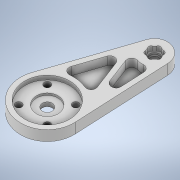
# Autodesk Inventor part: 足首_独立ピッチ_1_1
Saved by Autodesk Inventor 2020 (Build 240168000, 168)
## iProperties
Created: 2021-09-01
Part Number: 足首_独立ピッチ_1_1
Material: アルミニウム 2014-T4
Document SubType Name: Modeling
Designer: naoki
Density: 2.8 g/cm^3
Appearance: 滑らか - 淡い灰色
Author: naoki
Autodesk Inventor part; units mm, degrees
ref_plane "YZ Plane" through (0, 0, 0) normal (1, 0, 0) x (0, 1, 0)
ref_plane "XZ Plane" through (0, 0, 0) normal (0, 1, 0) x (-1, 0, 0)
ref_plane "XY Plane" through (0, 0, 0) normal (0, 0, 1) x (1, 0, 0)
derived "下半身全体像_1_1.ipt"
sketch "スケッチ1" plane through (0, 0, 0) normal (0, 0, 1) x (1, 0, 0)
  circle A0 centre (0, 0) radius 10.5 construction
  line L0 (0, 0) -> (-12, 0) construction
  arc A1 (0, 16) -> (-12, 10.583) centre (0, 0) ccw construction
  arc A2 (-12, -10.583) -> (0, -16) centre (0, 0) ccw construction
  line L1 (0, 16) -> (39.5, 16) construction
  line L2 (39.5, 16) -> (39.5, -16) construction
  line L3 (39.5, -16) -> (0, -16) construction
  circle A3 centre (1, 13.5) radius 1.35 projected
  circle A4 centre (1, -13.5) radius 1.35 projected
  circle A5 centre (28, 13.5) radius 1.35 projected
  circle A6 centre (28, -13.5) radius 1.35 projected
  line L4 (1, 13.5) -> (1, -13.5) construction
  line L5 (1, -13.5) -> (28, -13.5) construction
  line L6 (1, 13.5) -> (28, 13.5) construction
  line L7 (28, 13.5) -> (28, -13.5) construction
  line L8 (0, 0) -> (1, 0) construction
  line L9 (32, 120) -> (32, 20) construction
  line L10 (0, 0) -> (0, 0) construction
  circle A7 centre (32, 120) radius 4.05 projected
  line L11 (0, 140) -> (0, 40) construction
  circle A8 centre (0, 40) radius 4.05 projected
  line L12 (0, 0) -> (0, -100) construction
  line L13 (32, 20) -> (32, -80) construction
  line L14 (0, 0) -> (0, 40) construction
  circle A9 centre (32, 20) radius 6.5 construction
  line L15 (32, 23.5218) -> (35.05, 21.7609) construction
  line L16 (35.05, 21.7609) -> (35.05, 18.2391) construction
  line L17 (35.05, 18.2391) -> (32, 16.4782) construction
  line L18 (32, 16.4782) -> (28.95, 18.2391) construction
  line L19 (28.95, 18.2391) -> (28.95, 21.7609) construction
  line L20 (28.95, 21.7609) -> (32, 23.5218) construction
  line L21 (21.5, 152) -> (61, 152) construction
  line L22 (61, 152) -> (61, 100.5) construction
  line L23 (61, 100.5) -> (21.5, 100.5) construction
  line L24 (21.5, 100.5) -> (21.5, 152) construction
  line L25 (21.5, 140) -> (61, 140) construction
  line L26 (16, 150.5) -> (66.5, 150.5) construction
  line L27 (66.5, 150.5) -> (66.5, 129.5) construction
  line L28 (66.5, 129.5) -> (16, 129.5) construction
  line L29 (16, 129.5) -> (16, 150.5) construction
  circle A10 centre (0, 140) radius 10.5 construction
  line L30 (-13.5, 139) -> (13.5, 139) construction
  line L31 (13.5, 139) -> (13.5, 112) construction
  line L32 (13.5, 112) -> (-13.5, 112) construction
  line L33 (-13.5, 112) -> (-13.5, 139) construction
  circle A11 centre (-13.5, 139) radius 1.35 projected
  circle A12 centre (13.5, 139) radius 1.35 projected
  circle A13 centre (-13.5, 112) radius 1.35 projected
  circle A14 centre (13.5, 112) radius 1.35 projected
  line L34 (-12, 10.583) -> (-12, -10.583) construction
  circle A15 centre (0, -100) radius 4.05 construction
  circle A16 centre (32, -80) radius 4.05 construction
  circle A17 centre (0, -100) radius 10.5 construction
  line L35 (32, -80) -> (0, -100) construction
  line L36 (45, -60.5) -> (77.5, -60.5) construction
  line L37 (77.5, -60.5) -> (77.5, -112) construction
  line L38 (77.5, -112) -> (45, -112) construction
  line L39 (45, -112) -> (45, -60.5) construction
  line L40 (45, -100) -> (77.5, -100) construction
  line L41 (39.5, -89.5) -> (83, -89.5) construction
  line L42 (83, -89.5) -> (83, -110.5) construction
  line L43 (83, -110.5) -> (39.5, -110.5) construction
  line L44 (39.5, -110.5) -> (39.5, -89.5) construction
  line L45 (1, -86.5) -> (28, -86.5) construction
  line L46 (28, -86.5) -> (28, -113.5) construction
  line L47 (28, -113.5) -> (1, -113.5) construction
  line L48 (1, -113.5) -> (1, -86.5) construction
  circle A18 centre (1, -86.5) radius 1.35 construction
  circle A19 centre (1, -113.5) radius 1.35 construction
  circle A20 centre (28, -113.5) radius 1.35 construction
  circle A21 centre (28, -86.5) radius 1.35 construction
  circle A22 centre (32, 20) radius 4.05 projected
  circle A23 centre (32, 20) radius 4.05 projected
  line L49 (10.583, 152) -> (-10.583, 152) construction
  line L50 (16, 140) -> (16, 100.5) construction
  line L51 (16, 100.5) -> (-16, 100.5) construction
  line L52 (-16, 100.5) -> (-16, 140) construction
  arc A24 (16, 140) -> (10.583, 152) centre (0, 140) ccw construction
  arc A25 (-10.583, 152) -> (-16, 140) centre (0, 140) ccw construction
  line L53 (-12, -89.417) -> (-12, -110.583) construction
  line L54 (0, -84) -> (39.5, -84) construction
  line L55 (39.5, -84) -> (39.5, -116) construction
  line L56 (39.5, -116) -> (0, -116) construction
  arc A26 (0, -84) -> (-12, -89.417) centre (0, -100) ccw construction
  arc A27 (-12, -110.583) -> (0, -116) centre (0, -100) ccw construction
  circle A28 centre (-8.5, 0) radius 1.35 projected
  circle A29 centre (0, 0) radius 8.5 construction
  line L57 (35.05, 121.7609) -> (35.05, 118.2391) construction
  line L58 (35.05, 118.2391) -> (32, 116.4782) construction
  line L59 (32, 116.4782) -> (28.95, 118.2391) construction
  line L60 (28.95, 118.2391) -> (28.95, 121.7609) construction
  line L61 (28.95, 121.7609) -> (32, 123.5218) construction
  line L62 (32, 123.5218) -> (35.05, 121.7609) construction
  line L63 (0, 152) -> (0, 140) construction
  line L64 (0, 140) -> (0, 139) construction
  circle A30 centre (0, -100) radius 5.01
  circle A31 centre (0, -100) radius 12 construction
  circle A32 centre (-8.5, -100) radius 1.35
  line L65 (-24.9932, -100) -> (93.0564, -100) construction
  circle A33 centre (0, -100) radius 2.25
  circle A34 centre (0, -100) radius 12.5
  circle A35 centre (0, -100) radius 10.51
  circle A36 centre (0, -108.5) radius 1.35
  circle A37 centre (8.5, -100) radius 1.35
  circle A38 centre (0, -91.5) radius 1.35
  circle A39 centre (32, -80) radius 1.55
  circle A40 centre (32, -80) radius 2.25
  line L66 (-4.7001, -88.4173) -> (29.7439, -74.4403)
  line L67 (36.0089, -84.4642) -> (8.3518, -109.3004)
  circle A41 centre (32, -80) radius 6
  circle A42 centre (32, -80) radius 2.76 construction
  line L68 (33.5935, -82.76) -> (32.5435, -82.76)
  line L69 (30.4065, -82.76) -> (29.8815, -81.8507)
  line L70 (28.813, -80) -> (29.338, -79.0907)
  line L71 (30.4065, -77.24) -> (31.4565, -77.24)
  line L72 (33.5935, -77.24) -> (35.187, -80)
  line L73 (35.187, -80) -> (33.5935, -82.76)
  arc A43 (31.4565, -77.24) -> (29.8815, -78.1493) centre (30.9315, -78.1493) ccw
  line L74 (32, -80) -> (30.4065, -77.24) construction
  arc A44 (29.338, -79.0907) -> (29.338, -80.9093) centre (29.863, -80) ccw
  arc A45 (29.8815, -81.8507) -> (31.4565, -82.76) centre (30.9315, -81.8507) ccw
  arc A46 (32.5435, -82.76) -> (34.1185, -81.8507) centre (33.0685, -81.8507) ccw
  arc A47 (34.662, -80.9093) -> (34.662, -79.0907) centre (34.137, -80) ccw
  arc A48 (34.1185, -78.1493) -> (32.5435, -77.24) centre (33.0685, -78.1493) ccw
  line L75 (31.3452, -85.9642) -> (12.0618, -103.2808)
  line L76 (2.3365, -87.7203) -> (26.352, -77.9751)
  line L77 (26.734, -77.1244) -> (26.2459, -78.0181) construction
  line L78 (12.825, -102.5953) -> (10.9709, -105.9909) construction
  line L79 (26.2459, -78.0181) -> (12.825, -102.5953)
  line L80 (23.3185, -79.2061) -> (12.4661, -99.0797)
  line L81 (31.4565, -77.24) -> (32.5435, -77.24)
  line L82 (32.5435, -77.24) -> (33.5935, -77.24)
  line L83 (29.8815, -78.1493) -> (30.4065, -77.24)
  line L84 (29.338, -79.0907) -> (29.8815, -78.1493)
  line L85 (29.338, -80.9093) -> (28.813, -80)
  line L86 (29.8815, -81.8507) -> (29.338, -80.9093)
  line L87 (31.4565, -82.76) -> (30.4065, -82.76)
  line L88 (32.5435, -82.76) -> (31.4565, -82.76)
  point P0 (66.5, 140)
  point P1 (39.5, 0)
  point P2 (83, -100)
  point P3 (1, -100)
  point P4 (-12, -100)
  point P5 (39.5, -100)
  point P6 (83, -100)
  point P7 (34.3902, -81.38)
  point P8 (28.813, -80)
  point P9 (30.4065, -82.76)
  point P10 (33.5935, -82.76)
  point P11 (35.187, -80)
  point P12 (33.5935, -77.24)
  point P13 (34.662, -80.9093)
  point P14 (34.662, -79.0907)
  point P15 (34.1185, -78.1493)
  dimension "d5" = 17
  dimension "d60" = 5.52
  dimension "d2" = 10.02
  dimension "d15" = 8.5
  dimension "d48" = 4.5
  dimension "d49" = 25
  dimension "d50" = 21.02
  dimension "d51" = 2.7
  dimension "d54" = 360
  dimension "d56" = 3.1
  dimension "d58" = 4.5
  dimension "d59" = 6
  dimension "d61" = 2.1
  dimension "d64" = 360
  dimension "d68" = 2
  dimension "d69" = 2
  dimension "d71" = 2
  constraints: 48 end point, 29 point on circle, 18 centre point, 12 coincident, 11 tangent, 6 parallel, 6 point on line, 2 horizontal, 2 midpoint, 1 horizontal alignment, 1 perpendicular, 1 vertical, 60 other
  measures "d2" diameter of A30
  measures "d15" distance of A32.centre A15.centre
  measures "d48" diameter of A33
  measures "d49" diameter of A34
  measures "d50" diameter of A35
  measures "d51" diameter of A32
  measures "d56" diameter of A39
  measures "d58" diameter of A40
  measures "d59" radius of A41
  measures "d61" diameter of A43
  measures "d68" distance between parallel lines of L67 L75
  measures "d69" distance between parallel lines of L66 L76
  measures "d71" distance between parallel lines of L80 L79
extrude "押し出し5" add sketch "スケッチ1" along normal blind 1 contours A34 L76 L80 | L79 L76 A41 L75
extrude "押し出し6" add sketch "スケッチ1" along normal blind 2 contours A30 | A40
extrude "押し出し7" add sketch "スケッチ1" along normal blind 2.8 contours A46 L68 | L68 L88 L87 L69 L86 L85 L70 L84 L83 L71 L81 L82 L72 L73 | L73 A46 | A45 L87 | L73 A47 | A45 L69 | L72 A47 | A44 L85 | L72 A48 | A44 L70 | L82 A48 | A43 L83 | L71 A43
extrude "押し出し8" add sketch "スケッチ1" along normal blind 3 contours A35
extrude "押し出し9" add sketch "スケッチ1" along normal blind 5 contours A34 | A34 L80 L76 L79 L75 | L75 A41 L67 A34 | A34 L66 A41 L76 | A41
fillet "フィレット2" radius 2.1 7 edges at (23.3185, -79.2061, 3) (26.352, -77.9751, 3) (31.3452, -85.9642, 3) (12.825, -102.5953, 3) (12.4661, -99.0797, 3) (2.3365, -87.7203, 3) (26.2459, -78.0181, 3)
equation "\"d15\" = 0.5 * d5"
equation "\"d69\" = d68"
